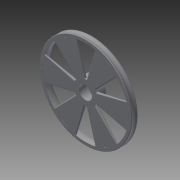
# Autodesk Inventor part: BackWheel
Saved by Autodesk Inventor 2014 SP1 (Build 180222100, 222)
## iProperties
Created: 2017-01-04
Part Number: BackWheel
Material: Generic
Document SubType Name: Modeling
Designer: danielsikar
Density: 1 g/cm^3
Appearance: Default
Author: danielsikar
Autodesk Inventor part; units mm, degrees
ref_plane "XZ Plane" through (0, 0, 0) normal (0, 1, 0) x (-1, 0, 0)
sketch "Sketch1" plane through (0, 0, 0) normal (0, 0, 1) x (1, 0, 0)
  line L0 (0, 0) -> (35, 0) construction
  line L1 (35, 3.8381) -> (35, -4.2783) construction
  line L2 (36.5, 4.6003) -> (36.5, -5.7654) construction
  line L3 (33.4599, 5) -> (40.8962, 5) construction
  line L4 (33.4599, 2.5) -> (40.8962, 2.5) construction
  arc A0 (35, 1.6177) -> (35, 1.3723) centre (36.5, 1.495) ccw
  arc A1 (36.5, 5) -> (36.5, 0) centre (37.8333, 2.5) ccw
  line L5 (36.5, 5) -> (33.1222, 5)
  line L6 (36.5, 0) -> (33.1222, 0)
  arc A2 (33.1222, 5) -> (33.1222, 0) centre (37.8333, 2.5) ccw
  arc A3 (35, -2.0185) -> (35.3235, -2.2059) centre (37.8333, 2.5) ccw
  line L7 (0, -7.9185) -> (0, 7.1531) projected
  dimension "d0" = 35
  dimension "d1" = 1.5
  dimension "d2" = 5
  dimension "d3" = 2.5
  constraints: 14 end point, 8 point on circle, 7 point on line, 4 centre point, 3 perpendicular, 1 horizontal, 1 parallel
  measures "d0" distance of L0.start L0.end
  measures "d1" distance from line of L2 L0.end
  measures "d2" distance between parallel lines of L3 L0
  measures "d3" distance between parallel lines of L4 L0
revolve "Revolution1" add sketch "Sketch1" angle 360 about axis through (0, -10, 0) along (0, 1, 0)
fillet "Fillet1" radius 0.5 2 edges at (-36.5, 5, 0) (-36.5, 0, 0)
sketch "Sketch2" plane through (0, 0, 0) normal (0, 1, 0) x (-1, 0, 0)
  circle A0 centre (0, 0) radius 6.25
  circle A1 centre (0, 0) radius 9
  dimension "d8" = 12.5
  dimension "d9" = 18
  constraints: 2 centre point, 2 coincident
  measures "d8" diameter of A0
  measures "d9" diameter of A1
extrude "Extrusion1" add sketch "Sketch2" along normal blind 7
ref_plane "Work Plane1" through (33, 0, 0) normal (1, 0, 0) x (0, 1, 0)
sketch "Sketch3" plane through (33, 0, 0) normal (1, 0, 0) x (0, 1, 0)
  line L0 (0.5, 10) -> (0.5, 10)
  line L1 (1, 9.5) -> (1, -9.5)
  line L2 (0.5, -10) -> (0.5, -10)
  line L3 (0, -9.5) -> (0, 9.5)
  arc A0 (1, 9.5) -> (0.5, 10) centre (0.5, 9.5) ccw
  arc A1 (0.5, 10) -> (0, 9.5) centre (0.5, 9.5) ccw
  arc A2 (0, -9.5) -> (0.5, -10) centre (0.5, -9.5) ccw
  arc A3 (0.5, -10) -> (1, -9.5) centre (0.5, -9.5) ccw
  line L4 (0, -35.1667) -> (0, 35.1667) projected
  point P0 (0, 0)
  point P1 (1, -10)
  point P2 (1, 10)
  point P3 (0, -10)
  dimension "d13" = 1
  dimension "d14" = 20
  dimension "d15" = 10
  dimension "d16" = 0.5
  dimension "d30" = 0
  constraints: 8 end point, 8 point on circle, 8 tangent, 6 point on line, 4 centre point, 3 equal radius, 2 parallel, 1 horizontal, 1 perpendicular
  measures "d13" distance of point (1, -10) point (0, -10)
  measures "d14" distance of point (1, 10) point (1, -10)
  measures "d15" distance from line of point (0, 0) L0
  measures "d16" radius of A0
  measures "d30" distance between parallel lines of L4 L3
ref_plane "Work Plane2" through (8, 0, 0) normal (1, 0, 0) x (0, 1, 0)
sketch "Sketch4" plane through (8, 0, 0) normal (1, 0, 0) x (0, 1, 0)
  line L0 (1, -4) -> (1, -4)
  line L1 (2, -3) -> (2, 3)
  line L2 (1, 4) -> (1, 4)
  line L3 (0, 3) -> (0, -3)
  arc A0 (1, 4) -> (0, 3) centre (1, 3) ccw
  arc A1 (2, 3) -> (1, 4) centre (1, 3) ccw
  arc A2 (0, -3) -> (1, -4) centre (1, -3) ccw
  arc A3 (1, -4) -> (2, -3) centre (1, -3) ccw
  point P0 (0, 0)
  point P1 (2, 4)
  point P2 (2, -4)
  point P3 (0, 4)
  dimension "d18" = 2
  dimension "d19" = 8
  dimension "d20" = 4
  dimension "d21" = 1
  dimension "d29" = 1
  constraints: 8 end point, 8 point on circle, 8 tangent, 6 point on line, 4 centre point, 2 equal radius, 2 parallel, 1 horizontal, 1 perpendicular
  measures "d18" distance of point (0, 4) point (2, 4)
  measures "d19" distance of point (2, 4) point (2, -4)
  measures "d20" distance from line of point (0, 0) L2
  measures "d21" radius of A0
  measures "d29" radius of A3
loft "Loft1" add profiles "Sketch3", "Sketch4"
pattern_circular "Circular Pattern1" count 6 over 360 about axis through (0, -10, 0) along (0, 1, 0) of "Loft1"
sketch "Sketch5" plane through (0, 0, 0) normal (0, 1, 0) x (-1, 0, 0)
  circle A0 centre (0, 0) radius 6.25
  circle A1 centre (0, 0) radius 5
  dimension "d31" = 12.5
  dimension "d32" = 10
  constraints: 2 centre point, 2 coincident
  measures "d31" diameter of A0
  measures "d32" diameter of A1
extrude "Extrusion2" add sketch "Sketch5" along normal blind 2
body "Solid1"
